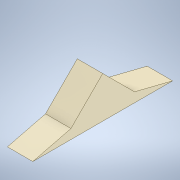
# Autodesk Inventor part: roof
Saved by Autodesk Inventor 2021.1 (Build 251245000, 245)
## iProperties
Created: 2020-03-27
Part Number: roof
Material: PET Plastic
Document SubType Name: Modeling
Designer: robst
Density: 1.541 g/cm^3
Appearance: Light Beige
Author: robst
Autodesk Inventor part; units mm, degrees
ref_plane "YZ Plane" through (0, 0, 0) normal (1, 0, 0) x (0, 1, 0)
ref_plane "XZ Plane" through (0, 0, 0) normal (0, 1, 0) x (-1, 0, 0)
ref_plane "XY Plane" through (0, 0, 0) normal (0, 0, 1) x (1, 0, 0)
sketch "Sketch1" plane through (0, 0, 0) normal (1, 0, 0) x (0, 1, 0)
  line L0 (0, 0) -> (914.4, 0)
  line L1 (914.4, 0) -> (0, 3657.6)
  line L2 (0, 3657.6) -> (0, 0)
  line L3 (914.4, 0) -> (3962.4, -3048)
  line L4 (3962.4, -3048) -> (914.4, -3048)
  line L5 (914.4, -3048) -> (914.4, 0)
  line L6 (0, 0) -> (0, -3048)
  line L7 (0, -3048) -> (914.4, -3048)
  dimension "rise" = 914.4
  dimension "run" = 3657.6
  dimension "roofAngle" = 14.036
  dimension "d9" = 45
  dimension "d10" = 3048
  constraints: 16 end point, 2 horizontal, 2 perpendicular, 2 vertical
  measures "rise" distance of L0.start L0.end
  measures "run" distance of L1.end L0.start
  measures "roofAngle" angle of L1 L2
  measures "d9" angle of L3 L5
  measures "d10" distance of L3.end L4.end
extrude "Extrusion1" add sketch "Sketch1" along normal mid plane 2438.4
mirror "Mirror1" about plane through (0, 0, -3048) normal (0, 0, -1) of "Extrusion1"
body "Solid1"
